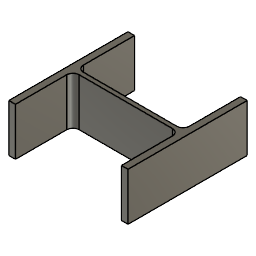
H-250×250×9×14 (Autodesk Fusion 360 design; units mm, degrees)
Autodesk Fusion 360 part; units mm, degrees
sketch "スケッチ1" plane through (0, 0, 0) normal (0, 0, 1) x (1, 0, 0)
  line L0 (0, 125) -> (0, -125)
  line L1 (250, -125) -> (250, 125)
  line L2 (236, -17.5) -> (236, -125)
  line L3 (14, -125) -> (14, -17.5)
  line L4 (0, -125) -> (14, -125)
  line L5 (236, -125) -> (250, -125)
  line L6 (223, 4.5) -> (27, 4.5)
  line L7 (27, -4.5) -> (223, -4.5)
  line L8 (14, 17.5) -> (14, 125)
  line L9 (14, 125) -> (0, 125)
  line L10 (236, 125) -> (236, 17.5)
  line L11 (250, 125) -> (236, 125)
  arc A0 (27, -4.5) -> (14, -17.5) centre (27, -17.5) ccw
  arc A1 (14, 17.5) -> (27, 4.5) centre (27, 17.5) ccw
  arc A2 (223, 4.5) -> (236, 17.5) centre (223, 17.5) ccw
  arc A3 (236, -17.5) -> (223, -4.5) centre (223, -17.5) ccw
extrude "押し出し1" add sketch "スケッチ1" along normal blind 100
